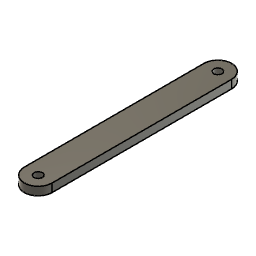
Robotica v10 (Autodesk Fusion 360 archive; units mm, degrees)
design "Double Door Opener 1"
Autodesk Fusion 360 part; units mm, degrees
sketch "Sketch1" plane through (0, 0, 0) normal (0, 1, 0) x (1, 0, 0)
  line L0 (5, 32.5) -> (-5, 32.5)
  line L1 (-5, 32.5) -> (-5, -32.5)
  line L2 (-5, -32.5) -> (5, -32.5)
  line L3 (5, -32.5) -> (5, 32.5)
  line L4 (5, 32.5) -> (-5, -32.5) construction
  line L5 (-5, 32.5) -> (5, -32.5) construction
  arc A0 (5, 32.5) -> (-5, 32.5) centre (0, 32.5) ccw
  line L6 (-5, 0) -> (5, 0) construction
  circle A1 centre (0, 32.5) radius 1.5
  arc A2 (-5, -32.5) -> (5, -32.5) centre (0, -32.5) ccw
  circle A3 centre (0, -32.5) radius 1.5
  dimension "d1" = 10
  dimension "d2" = 65
  dimension "d3" = 3
  constraint horizontal L0
  constraint perpendicular L0 L1
  constraint parallel L0 L2
  constraint parallel L1 L3
  constraint coincident L4 origin
  constraint coincident L5 origin
  constraint tangent L3 A0
  constraint midpoint L1 L6.start
  constraint midpoint L3 L6.end
  constraint concentric A0 A1
  constraint symmetric L0.start L6 L2.end
  constraint symmetric L0.end L6 L1.end
  constraint symmetric A0 L6 A2
  constraint symmetric L6 A1 A3
  measures "d1" distance of L1 L3
  measures "d2" distance of L0.end L1.end
  measures "d3" diameter of A1
extrude "Extrude1" add sketch "Sketch1" along normal blind 3 contours L0 L1 L2 L3 A1 A3 | L0 A0 A1 | L2 A2 A3

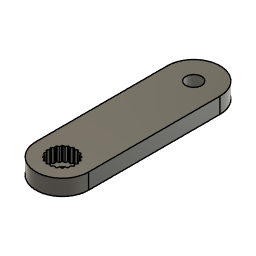
design "Double Door Opener 2"
Autodesk Fusion 360 part; units mm, degrees
sketch "Sketch1" plane through (0, 0, 0) normal (0, 1, 0) x (1, 0, 0)
  line L0 (5, 12.5) -> (-5, 12.5)
  line L1 (-5, 12.5) -> (-5, -12.5)
  line L2 (-5, -12.5) -> (5, -12.5)
  line L3 (5, -12.5) -> (5, 12.5)
  line L4 (5, 12.5) -> (-5, -12.5) construction
  line L5 (-5, 12.5) -> (5, -12.5) construction
  arc A0 (5, 12.5) -> (-5, 12.5) centre (0, 12.5) ccw
  line L6 (-5, 0) -> (5, 0) construction
  circle A1 centre (0, 12.5) radius 1.5
  arc A2 (-5, -12.5) -> (5, -12.5) centre (0, -12.5) ccw
  circle A3 centre (0, -12.5) radius 1.5
  dimension "d1" = 10
  dimension "d2" = 25
  dimension "d3" = 3
  constraint horizontal L0
  constraint perpendicular L0 L1
  constraint parallel L0 L2
  constraint parallel L1 L3
  constraint coincident L4 origin
  constraint coincident L5 origin
  constraint tangent L3 A0
  constraint midpoint L1 L6.start
  constraint midpoint L3 L6.end
  constraint concentric A0 A1
  constraint symmetric L0.start L6 L2.end
  constraint symmetric L0.end L6 L1.end
  constraint symmetric A0 L6 A2
  constraint symmetric L6 A1 A3
  measures "d1" distance of L1 L3
  measures "d2" distance of L0.end L1.end
  measures "d3" diameter of A1
extrude "Extrude1" add sketch "Sketch1" along normal blind 3 contours L0 L1 L2 L3 A1 A3 | L0 A0 A1 | L2 A2 A3 | L2 A3 | L2 A3
sketch "Boceto2" plane through (0, 3, 0) normal (0, 1, 0) x (-1, 0, 0)
  circle A0 centre (0, -12.5) radius 1.5
  arc A1 (5, 12.5) -> (-5, 12.5) centre (0, 12.5) ccw
  line L0 (-5, 12.5) -> (-5, -12.5)
  arc A2 (-5, -12.5) -> (5, -12.5) centre (0, -12.5) ccw
  line L1 (5, -12.5) -> (5, 12.5)
  circle A3 centre (0, 12.5) radius 2.63
  line L2 (0, 9.87) -> (0, 15.13) construction
  line L3 (0, 10.1418) -> (0.322, 9.8898)
  line L4 (0, 10.1418) -> (-0.322, 9.8898)
  line L5 (0.7287, 10.2572) -> (1.1128, 10.117)
  line L6 (0.7287, 10.2572) -> (0.5004, 9.918)
  line L7 (1.3861, 10.5922) -> (1.7947, 10.5776)
  line L8 (1.3861, 10.5922) -> (1.2737, 10.199)
  line L9 (1.9078, 11.1139) -> (2.301, 11.2263)
  line L10 (1.9078, 11.1139) -> (1.9224, 10.7053)
  line L11 (2.2428, 11.7713) -> (2.582, 11.9996)
  line L12 (2.2428, 11.7713) -> (2.383, 11.3872)
  line L13 (2.3582, 12.5) -> (2.6102, 12.822)
  line L14 (2.3582, 12.5) -> (2.6102, 12.178)
  line L15 (2.2428, 13.2287) -> (2.383, 13.6128)
  line L16 (2.2428, 13.2287) -> (2.582, 13.0004)
  line L17 (1.9078, 13.8861) -> (1.9224, 14.2947)
  line L18 (1.9078, 13.8861) -> (2.301, 13.7737)
  line L19 (1.3861, 14.4078) -> (1.2737, 14.801)
  line L20 (1.3861, 14.4078) -> (1.7947, 14.4224)
  line L21 (0.7287, 14.7428) -> (0.5004, 15.082)
  line L22 (0.7287, 14.7428) -> (1.1128, 14.883)
  line L23 (0, 14.8582) -> (-0.322, 15.1102)
  line L24 (0, 14.8582) -> (0.322, 15.1102)
  line L25 (-0.7287, 14.7428) -> (-1.1128, 14.883)
  line L26 (-0.7287, 14.7428) -> (-0.5004, 15.082)
  line L27 (-1.3861, 14.4078) -> (-1.7947, 14.4224)
  line L28 (-1.3861, 14.4078) -> (-1.2737, 14.801)
  line L29 (-1.9078, 13.8861) -> (-2.301, 13.7737)
  line L30 (-1.9078, 13.8861) -> (-1.9224, 14.2947)
  line L31 (-2.2428, 13.2287) -> (-2.582, 13.0004)
  line L32 (-2.2428, 13.2287) -> (-2.383, 13.6128)
  line L33 (-2.3582, 12.5) -> (-2.6102, 12.178)
  line L34 (-2.3582, 12.5) -> (-2.6102, 12.822)
  line L35 (-2.2428, 11.7713) -> (-2.383, 11.3872)
  line L36 (-2.2428, 11.7713) -> (-2.582, 11.9996)
  line L37 (-1.9078, 11.1139) -> (-1.9224, 10.7053)
  line L38 (-1.9078, 11.1139) -> (-2.301, 11.2263)
  line L39 (-1.3861, 10.5922) -> (-1.2737, 10.199)
  line L40 (-1.3861, 10.5922) -> (-1.7947, 10.5776)
  line L41 (-0.7287, 10.2572) -> (-0.5004, 9.918)
  line L42 (-0.7287, 10.2572) -> (-1.1128, 10.117)
  dimension "d6" = 5.26
  dimension "d7" = 0.252
  dimension "d8" = 0.322
  dimension "d10" = 360
  constraint concentric A1 A3
  constraint coincident A3 L2.start
  constraint coincident A3 L2.end
  constraint parallel L1 L2
  constraint coincident L2 L3.start
  constraint coincident A3 L3.end
  constraint coincident A1.centre L2
  constraint symmetric L2 L3.start L4.start
  constraint symmetric L2 L3.end L4.end
  measures "d6" diameter of A3
  measures "d7" vertical distance of L3.start L3.end
  measures "d8" horizontal distance of L3.start L3.end
extrude "Extruir2" cut sketch "Boceto2" against normal blind 2.6 contours A3 L3 L4 L5 L6 L7 L8 L9 L10 L11 L12 L13 L14 L15 L16 L17 L18 L19 L20 L21 L22 L23 L24 L25 L26 L27 L28 L29 L30 L31 L32 L33 L34 L35 L36 L37 L38 L39 L40 L41 L42
sketch "Boceto3" plane through (0, 0.4, 0) normal (0, 1, 0) x (-1, 0, 0)
  arc A0 (-0.5004, 9.918) -> (-0.322, 9.8898) centre (0, 12.5) ccw
  line L0 (-0.322, 9.8898) -> (0, 10.1418)
  line L1 (0, 10.1418) -> (0.322, 9.8898)
  arc A1 (0.322, 9.8898) -> (0.5004, 9.918) centre (0, 12.5) ccw
  line L2 (0.5004, 9.918) -> (0.7287, 10.2572)
  line L3 (0.7287, 10.2572) -> (1.1128, 10.117)
  arc A2 (1.1128, 10.117) -> (1.2737, 10.199) centre (0, 12.5) ccw
  line L4 (1.2737, 10.199) -> (1.3861, 10.5922)
  line L5 (1.3861, 10.5922) -> (1.7947, 10.5776)
  arc A3 (1.7947, 10.5776) -> (1.9224, 10.7053) centre (0, 12.5) ccw
  line L6 (1.9224, 10.7053) -> (1.9078, 11.1139)
  line L7 (1.9078, 11.1139) -> (2.301, 11.2263)
  arc A4 (2.301, 11.2263) -> (2.383, 11.3872) centre (0, 12.5) ccw
  line L8 (2.383, 11.3872) -> (2.2428, 11.7713)
  line L9 (2.2428, 11.7713) -> (2.582, 11.9996)
  arc A5 (2.582, 11.9996) -> (2.6102, 12.178) centre (0, 12.5) ccw
  line L10 (2.6102, 12.178) -> (2.3582, 12.5)
  line L11 (2.3582, 12.5) -> (2.6102, 12.822)
  arc A6 (2.6102, 12.822) -> (2.582, 13.0004) centre (0, 12.5) ccw
  line L12 (2.582, 13.0004) -> (2.2428, 13.2287)
  line L13 (2.2428, 13.2287) -> (2.383, 13.6128)
  arc A7 (2.383, 13.6128) -> (2.301, 13.7737) centre (0, 12.5) ccw
  line L14 (2.301, 13.7737) -> (1.9078, 13.8861)
  line L15 (1.9078, 13.8861) -> (1.9224, 14.2947)
  arc A8 (1.9224, 14.2947) -> (1.7947, 14.4224) centre (0, 12.5) ccw
  line L16 (1.7947, 14.4224) -> (1.3861, 14.4078)
  line L17 (1.3861, 14.4078) -> (1.2737, 14.801)
  arc A9 (1.2737, 14.801) -> (1.1128, 14.883) centre (0, 12.5) ccw
  line L18 (1.1128, 14.883) -> (0.7287, 14.7428)
  line L19 (0.7287, 14.7428) -> (0.5004, 15.082)
  arc A10 (0.5004, 15.082) -> (0.322, 15.1102) centre (0, 12.5) ccw
  line L20 (0.322, 15.1102) -> (0, 14.8582)
  line L21 (0, 14.8582) -> (-0.322, 15.1102)
  arc A11 (-0.322, 15.1102) -> (-0.5004, 15.082) centre (0, 12.5) ccw
  line L22 (-0.5004, 15.082) -> (-0.7287, 14.7428)
  line L23 (-0.7287, 14.7428) -> (-1.1128, 14.883)
  arc A12 (-1.1128, 14.883) -> (-1.2737, 14.801) centre (0, 12.5) ccw
  line L24 (-1.2737, 14.801) -> (-1.3861, 14.4078)
  line L25 (-1.3861, 14.4078) -> (-1.7947, 14.4224)
  arc A13 (-1.7947, 14.4224) -> (-1.9224, 14.2947) centre (0, 12.5) ccw
  line L26 (-1.9224, 14.2947) -> (-1.9078, 13.8861)
  line L27 (-1.9078, 13.8861) -> (-2.301, 13.7737)
  arc A14 (-2.301, 13.7737) -> (-2.383, 13.6128) centre (0, 12.5) ccw
  line L28 (-2.383, 13.6128) -> (-2.2428, 13.2287)
  line L29 (-2.2428, 13.2287) -> (-2.582, 13.0004)
  arc A15 (-2.582, 13.0004) -> (-2.6102, 12.822) centre (0, 12.5) ccw
  line L30 (-2.6102, 12.822) -> (-2.3582, 12.5)
  line L31 (-2.3582, 12.5) -> (-2.6102, 12.178)
  arc A16 (-2.6102, 12.178) -> (-2.582, 11.9996) centre (0, 12.5) ccw
  line L32 (-2.582, 11.9996) -> (-2.2428, 11.7713)
  line L33 (-2.2428, 11.7713) -> (-2.383, 11.3872)
  arc A17 (-2.383, 11.3872) -> (-2.301, 11.2263) centre (0, 12.5) ccw
  line L34 (-2.301, 11.2263) -> (-1.9078, 11.1139)
  line L35 (-1.9078, 11.1139) -> (-1.9224, 10.7053)
  arc A18 (-1.9224, 10.7053) -> (-1.7947, 10.5776) centre (0, 12.5) ccw
  line L36 (-1.7947, 10.5776) -> (-1.3861, 10.5922)
  line L37 (-1.3861, 10.5922) -> (-1.2737, 10.199)
  arc A19 (-1.2737, 10.199) -> (-1.1128, 10.117) centre (0, 12.5) ccw
  line L38 (-1.1128, 10.117) -> (-0.7287, 10.2572)
  line L39 (-0.7287, 10.2572) -> (-0.5004, 9.918)
  circle A20 centre (0, 12.5) radius 1.375
  dimension "d13" = 2.75
  constraint concentric A0 A20
  measures "d13" diameter of A20
extrude "Extruir3" cut sketch "Boceto3" against normal blind 0.5 contours A20

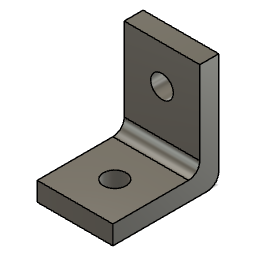
design "Double Door Opener 3"
Autodesk Fusion 360 part; units mm, degrees
sketch "Sketch1" plane through (0, 0, 0) normal (0, 1, 0) x (1, 0, 0)
  line L0 (5, 6.5) -> (-5, 6.5)
  line L1 (-5, 6.5) -> (-5, -6.5)
  line L2 (-5, -6.5) -> (5, -6.5)
  line L3 (5, -6.5) -> (5, 6.5)
  line L4 (5, 6.5) -> (-5, -6.5) construction
  line L5 (-5, 6.5) -> (5, -6.5) construction
  circle A0 centre (0, -1.25) radius 1.5
  dimension "d1" = 13
  dimension "d2" = 10
  dimension "d21" = 3
  dimension "d22" = 1.25
  constraint horizontal L0
  constraint perpendicular L0 L1
  constraint parallel L0 L2
  constraint parallel L1 L3
  constraint coincident L4 origin
  constraint coincident L5 origin
  measures "d1" distance of L0.end L1.end
  measures "d2" distance of L0.start L0.end
  measures "d21" diameter of A0
  measures "d22" distance of origin A0.centre
extrude "Extrude1" add sketch "Sketch1" along normal blind 2.5
sketch "Sketch3" plane through (0, 0, 0) normal (0, 1, 0) x (1, 0, 0)
  line L0 (-5, 5) -> (5, 5)
  line L1 (5, 5) -> (5, 7.5)
  line L2 (5, 7.5) -> (-5, 7.5)
  line L3 (-5, 7.5) -> (-5, 5)
  dimension "d10" = 2.5
  dimension "d11" = 10
  dimension "d12" = 5
  dimension "d13" = 5
  constraint horizontal L0
  constraint vertical L1
  constraint horizontal L2
  constraint vertical L3
  measures "d10" distance of L0.start L2.end
  measures "d11" distance of L1.end L2.end
  measures "d12" vertical distance of origin L0.end
  measures "d13" horizontal distance of origin L0.start
extrude "Extrude3" add sketch "Sketch3" along normal blind 15
sketch "Sketch5" plane through (0, 0, -5) normal (0, 0, 1) x (1, 0, 0)
  line L0 (5, 2.5) -> (5, 15)
  line L1 (5, 15) -> (-5, 15)
  line L2 (-5, 15) -> (-5, 2.5)
  circle A0 centre (0, 10) radius 1.5
  line L3 (-5, 2.5) -> (5, 2.5)
  dimension "d16" = 5
  dimension "d17" = 3
  constraint vertical origin A0.centre
  measures "d16" vertical distance of L1.end A0.centre
  measures "d17" diameter of A0
extrude "Extrude4" cut sketch "Sketch5" against normal blind 45 contours A0
fillet "Fillet1" radius 1.5 2 edges at (0, 2.5, -5) (0, 0, -7.5)
